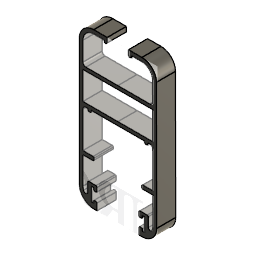
Cerco (Autodesk Fusion 360 design; units mm, degrees)
part number: 2025-12-27-23-45-21-865
Autodesk Fusion 360 part; units mm, degrees
note: some values were not read from the file. Set by a fixed rule: which sketch regions a step uses.
sketch "Boceto2" plane through (0, 0, 0) normal (0, 1, 0) x (1, 0, 0)
  line L0 (7.5, 0) -> (9.2213, 0)
  line L1 (14.5, -80.7) -> (7.5, -80.7)
  line L2 (0, -73.2) -> (0, -7.5)
  arc A0 (0, -73.2) -> (7.5, -80.7) centre (7.5, -73.2) ccw
  arc A1 (7.5, 0) -> (0, -7.5) centre (7.5, -7.5) ccw
  line L3 (12.7, -78.7828) -> (7.5, -78.7828)
  arc A2 (1.9172, -73.2) -> (7.5, -78.7828) centre (7.5, -73.2) ccw
  line L4 (7.5, -3.5523) -> (7.5, -2.6)
  line L5 (7.5, -2.6) -> (6.3, -2.6)
  line L6 (6.3, -2.6) -> (6.3, -9.6)
  line L7 (6.3, -9.6) -> (7.5, -9.6)
  line L8 (7.5, -9.6) -> (7.5, -8.5)
  line L9 (9.2213, -8.5) -> (9.2213, -10.6)
  line L10 (8.7213, -11.1) -> (4.9, -11.1)
  line L11 (4.4, -10.6) -> (4.4, -5.7)
  arc A3 (4.4, -5.7) -> (2.8546, -5.0381) centre (3.3076, -6.1153) ccw
  arc A4 (4.4, -5.7) -> (2.1854, -5.7893) centre (3.3076, -6.1153) ccw
  arc A5 (2.1854, -5.7893) -> (1.9172, -7.5) centre (7.5062, -7.5) ccw
  arc A6 (9.2213, -8.5) -> (7.5, -8.5) centre (8.3607, -9.2707) ccw
  arc A7 (7.5, -3.5523) -> (9.2213, -3.5523) centre (8.3607, -3.072) ccw
  line L12 (9.2213, -3.5523) -> (9.2213, 0)
  line L13 (20.1126, -1.9172) -> (20.115, -1.9172)
  line L14 (1.9172, -21.6025) -> (7.2, -21.6025)
  line L15 (7.7, -22.1025) -> (7.7, -23)
  line L16 (7.2, -23.5) -> (1.9172, -23.5)
  line L17 (1.9172, -45.6046) -> (20.0634, -45.6046)
  line L18 (20.0634, -43.7426) -> (20.0634, -43.7426)
  line L19 (20.036, -60.0002) -> (20.036, -60.0234)
  line L20 (20.036, -61.8138) -> (3.4172, -61.8138)
  line L21 (14.5, -80.7) -> (14.5, -78.7828)
  line L22 (1.9172, -21.6025) -> (1.9172, -7.5)
  arc A8 (7.2, -23.5) -> (7.7, -23) centre (7.2, -23) ccw
  arc A9 (7.7, -22.1025) -> (7.2, -21.6025) centre (7.2, -22.1025) ccw
  line L23 (1.9172, -42.2426) -> (1.9172, -23.5)
  arc A10 (1.9172, -42.2426) -> (3.4172, -43.7426) centre (3.4172, -42.2426) ccw
  line L24 (6.2895, -43.7426) -> (6.2895, -43.415)
  line L25 (4.4317, -43.415) -> (4.4317, -43.7426)
  arc A11 (6.2895, -43.415) -> (4.4317, -43.415) centre (5.3606, -43.415) ccw
  line L26 (20.0634, -43.7426) -> (6.2895, -43.7426)
  line L27 (4.4317, -43.7426) -> (3.4172, -43.7426)
  line L28 (1.9172, -73.2) -> (1.9172, -63.3138)
  line L29 (1.9172, -60.0002) -> (1.9172, -45.6046)
  arc A12 (3.4172, -61.8138) -> (1.9172, -63.3138) centre (3.4172, -63.3138) ccw
  line L30 (12.9, -78.5828) -> (12.9, -78.2)
  line L31 (14.5, -78.2) -> (14.5, -78.7828)
  arc A13 (14.5, -78.2) -> (12.9, -78.2) centre (13.7, -78.34) ccw
  arc A14 (4.4, -10.6) -> (4.9, -11.1) centre (4.9, -10.6) ccw
  arc A15 (8.7213, -11.1) -> (9.2213, -10.6) centre (8.7213, -10.6) ccw
  arc A16 (12.7, -78.7828) -> (12.9, -78.5828) centre (12.7, -78.5828) ccw
  line L32 (32.4735, -22.1342) -> (32.4712, -23.0317)
  line L33 (35.8029, -10.6401) -> (35.8154, -5.7401)
  arc A17 (36.701, -43.7851) -> (38.2048, -42.289) centre (36.7048, -42.2851) ccw
  line L34 (38.1594, -60.0465) -> (38.1962, -45.651)
  line L35 (33.8286, -43.7778) -> (33.8295, -43.4502)
  arc A18 (35.6873, -43.4549) -> (33.8295, -43.4502) centre (34.7584, -43.4526) ccw
  line L36 (32.7209, -3.5846) -> (32.7233, -2.6322)
  line L37 (35.6864, -43.7825) -> (36.701, -43.7851)
  line L38 (32.9699, -23.5329) -> (38.2527, -23.5464)
  line L39 (40.0429, -73.2512) -> (40.2108, -7.5514)
  line L40 (38.2048, -42.289) -> (38.2527, -23.5464)
  arc A19 (32.4712, -23.0317) -> (32.9699, -23.5329) centre (32.9712, -23.0329) ccw
  line L41 (35.6873, -43.4549) -> (35.6864, -43.7825)
  arc A20 (37.3625, -5.0822) -> (35.8154, -5.7401) centre (36.9067, -6.1583) ccw
  line L42 (30.9869, -8.5278) -> (30.9816, -10.6278)
  line L43 (27.1292, -78.601) -> (27.1301, -78.2182)
  arc A21 (38.2936, -7.5465) -> (38.0298, -5.8351) centre (32.7046, -7.5322) ccw
  line L44 (25.5301, -78.2141) -> (25.5286, -78.7969)
  line L45 (32.73, -0.0322) -> (31.0086, -0.0278)
  arc A22 (40.2108, -7.5514) -> (32.73, -0.0322) centre (32.7108, -7.5322) ccw
  arc A23 (35.3016, -11.1388) -> (35.8029, -10.6401) centre (35.3029, -10.6388) ccw
  arc A24 (32.5237, -80.732) -> (40.0429, -73.2512) centre (32.5429, -73.232) ccw
  arc A25 (32.9748, -21.6355) -> (32.4735, -22.1342) centre (32.9735, -22.1355) ccw
  line L46 (32.7054, -9.6322) -> (32.7082, -8.5322)
  arc A26 (30.9816, -10.6278) -> (31.4803, -11.1291) centre (31.4816, -10.6291) ccw
  line L47 (33.9233, -2.6353) -> (33.9054, -9.6353)
  line L48 (27.3286, -78.8015) -> (32.5286, -78.8148)
  arc A27 (38.0298, -5.8351) -> (35.8154, -5.7401) centre (36.9067, -6.1583) ccw
  arc A28 (38.151, -63.3601) -> (36.6548, -61.8563) centre (36.651, -63.3563) ccw
  arc A29 (30.9996, -3.5802) -> (32.7209, -3.5846) centre (31.8615, -3.102) ccw
  line L49 (30.9996, -3.5802) -> (31.0086, -0.0278)
  arc A30 (32.5286, -78.8148) -> (38.1257, -73.2463) centre (32.5429, -73.232) ccw
  line L50 (38.1257, -73.2463) -> (38.151, -63.3601)
  line L51 (38.2576, -21.649) -> (38.2936, -7.5465)
  line L52 (31.4803, -11.1291) -> (35.3016, -11.1388)
  line L53 (25.5237, -80.7141) -> (25.5286, -78.7969)
  arc A31 (27.1292, -78.601) -> (27.3286, -78.8015) centre (27.3292, -78.6015) ccw
  line L54 (32.7233, -2.6322) -> (33.9233, -2.6353)
  line L55 (33.9054, -9.6353) -> (32.7054, -9.6322)
  arc A32 (32.7082, -8.5322) -> (30.9869, -8.5278) centre (31.8456, -9.3007) ccw
  line L56 (38.2576, -21.649) -> (32.9748, -21.6355)
  line L57 (25.5237, -80.7141) -> (32.5237, -80.732)
  arc A33 (27.1301, -78.2182) -> (25.5301, -78.2141) centre (26.3298, -78.3561) ccw
  line L58 (20.0548, -43.7426) -> (33.8286, -43.7778)
  line L59 (38.1962, -45.651) -> (20.05, -45.6046)
  line L60 (20.036, -61.8138) -> (36.6548, -61.8563)
  line L61 (1.9172, -60.0002) -> (38.1594, -60.0465)
  line L62 (20.036, -61.8138) -> (20.0119, -80.7) construction
  line L63 (20.115, 0) -> (20.0591, -43.7426) construction
  line L64 (20.0567, -45.6046) -> (20.0383, -60.0234) construction
  point P0 (0, -80.7)
  point P1 (40.0237, -80.7511)
  point P2 (40.2299, -0.0514)
  point P3 (40.2299, -0.0514)
  dimension "d10" = 80.7
  dimension "d12" = 7.5
  dimension "d14" = 0.5
  dimension "d15" = 1.5
  dimension "d16" = 1.5
  dimension "d17" = 0.5
  dimension "d18" = 0.2
  constraint horizontal L0
  constraint horizontal L1
  constraint vertical L2
  constraint coincident P0 L1
  constraint coincident P0 L2
  constraint tangent L1 A0
  constraint tangent L2 A0
  constraint coincident origin L0
  constraint coincident origin L2
  constraint tangent L0 A1
  constraint tangent L2 A1
  constraint equal A0 A1
  constraint perpendicular L4 L5
  constraint perpendicular L4 L7
  constraint perpendicular L7 L8
  constraint perpendicular L5 L9
  constraint perpendicular L9 L10
  constraint perpendicular L10 L11
  constraint concentric A0 A2
  constraint tangent L3 A2
  constraint tangent A2 L28
  constraint concentric A3 A4
  constraint tangent A5 L28
  constraint coincident L13.start L63
  constraint horizontal L14
  constraint vertical L15
  constraint horizontal L16
  constraint coincident L14.start L28
  constraint horizontal L17
  constraint vertical L18
  constraint horizontal L26
  constraint vertical L19
  constraint horizontal L20
  constraint coincident L20.start L63
  constraint coincident L29.start L28
  constraint perpendicular L3 L21
  constraint collinear L22 L28
  constraint tangent L15 A8
  constraint tangent L16 A8
  constraint tangent L14 A9
  constraint tangent L15 A9
  constraint equal A8 A9
  constraint collinear L23 L28
  constraint tangent A10 L26
  constraint tangent L23 A10
  constraint vertical L24
  constraint vertical L25
  constraint coincident L25.end L26
  constraint collinear L26 L27
  constraint collinear L28 L29
  constraint tangent L20 A12
  constraint tangent L28 A12
  constraint vertical L30
  constraint vertical L31
  constraint tangent L10 A14
  constraint tangent L11 A14
  constraint tangent L9 A15
  constraint tangent L10 A15
  constraint equal A14 A15
  constraint tangent L30 A16
  constraint tangent L3 A16
  constraint symmetric origin P3 L63
  constraint symmetric P0 P1 L63
  constraint symmetric L1.end A24.start L63
  constraint symmetric L2.start L39.start L63
  constraint symmetric A0 A24 L63
  constraint symmetric L0.start L45.start L63
  constraint symmetric L2.end L39.end L63
  constraint symmetric A1 A22 L63
  constraint symmetric L3.end L48.end L63
  constraint symmetric A2.start A30.end L63
  constraint symmetric A2 A30 L63
  constraint symmetric A5.end A21.start L63
  constraint symmetric A7.end A29.start L63
  constraint symmetric L4.start L36.start L63
  constraint symmetric L4.end L36.end L63
  constraint symmetric L5.end L47.start L63
  constraint symmetric L6.end L47.end L63
  constraint symmetric L7.end L46.start L63
  constraint symmetric L8.end L46.end L63
  constraint symmetric L9.start L42.start L63
  constraint symmetric L11.end L33.end L63
  constraint symmetric A3 A20 L63
  constraint symmetric A3.end A20.start L63
  constraint symmetric A4 A27 L63
  constraint symmetric A4.end A21.end L63
  constraint symmetric A5 A21 L63
  constraint symmetric A6 A32 L63
  constraint symmetric A7 A29 L63
  constraint symmetric L0.end L45.end L63
  constraint symmetric L14.start L51.start L63
  constraint symmetric L16.end L38.end L63
  constraint symmetric L17.start L34.end L63
  constraint symmetric L17.end L59.end L63
  constraint symmetric L18.start L58.start L63
  constraint symmetric L29.start L34.start L63
  constraint symmetric L20.start L60.start L63
  constraint symmetric L1.start L53.start L63
  constraint symmetric L21.end L44.end L63
  constraint symmetric L15.end L32.end L63
  constraint symmetric L16.start L38.start L63
  constraint symmetric A8 A19 L63
  constraint symmetric L14.end A25.start L63
  constraint symmetric L15.start L32.start L63
  constraint symmetric A9 A25 L63
  constraint symmetric A10.end A17.start L63
  constraint symmetric L23.start A17.end L63
  constraint symmetric A10 A17 L63
  constraint symmetric L25.end L37.start L63
  constraint symmetric L24.start L35.start L63
  constraint symmetric L24.end L35.end L63
  constraint symmetric L25.start A18.start L63
  constraint symmetric A11 A18 L63
  constraint symmetric L20.end A28.end L63
  constraint symmetric L28.end A28.start L63
  constraint symmetric A12 A28 L63
  constraint symmetric L30.end L43.end L63
  constraint symmetric L31.start L44.start L63
  constraint symmetric A13 A33 L63
  constraint symmetric L10.end A23.start L63
  constraint symmetric L11.start L33.start L63
  constraint symmetric A14 A23 L63
  constraint symmetric L9.end L42.end L63
  constraint symmetric L10.start A26.end L63
  constraint symmetric A15 A26 L63
  constraint symmetric L30.start L43.start L63
  constraint symmetric L3.start L48.start L63
  constraint symmetric A16 A31 L63
  constraint coincident L61 L64.end
  constraint collinear L62 L63
  constraint coincident L61 L19.end
  constraint coincident L26 L63.end
  constraint coincident L17 L64.start
  constraint collinear L63 L64
  constraint coincident L58 L18.start
  measures "d10" distance of origin P0
  measures "d12" radius of A0
  measures "d14" radius of A8
  measures "d15" radius of A10
  measures "d16" radius of A12
  measures "d17" radius of A14
  measures "d18" radius of A16
extrude "Extruir1" add sketch "Boceto2" along normal blind 10
equation "d19 = L"
equation "L = 10 mm"
